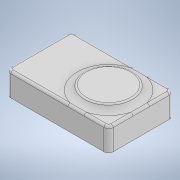
# Autodesk Inventor part: Black_Keyboard_Button
Saved by Autodesk Inventor 2021 (Build 250183000, 183)
## iProperties
Created: 2020-06-05
Part Number: Black_Keyboard_Button
Material: Generic
Document SubType Name: Modeling
Designer: ameli
Density: 1 g/cm^3
Appearance: Default
Author: ameli
Autodesk Inventor part; units mm, degrees
ref_plane "YZ Plane" through (0, 0, 0) normal (1, 0, 0) x (0, 1, 0)
ref_plane "XZ Plane" through (0, 0, 0) normal (0, 1, 0) x (-1, 0, 0)
ref_plane "XY Plane" through (0, 0, 0) normal (0, 0, 1) x (1, 0, 0)
sketch "Sketch1" plane through (0, 0, 0) normal (0, 1, 0) x (-1, 0, 0)
  line L0 (11, 7) -> (-11, 7)
  line L1 (-11, 7) -> (-11, -7)
  line L2 (-11, -7) -> (11, -7)
  line L3 (11, -7) -> (11, 7)
  point P0 (0, 0)
  dimension "d0" = 22
  dimension "d1" = 14
  dimension "d2" = 11
  dimension "d3" = 7
  constraints: 8 end point, 2 parallel, 1 horizontal, 1 perpendicular
  measures "d0" distance of L1.end L2.end
  measures "d1" distance of L2.end L0.start
  measures "d2" distance from line of point (0, 0) L3
  measures "d3" distance from line of point (0, 0) L2
extrude "Extrusion1" add sketch "Sketch1" along normal blind 5
sketch "Sketch2" plane through (0, 5, 0) normal (0, 1, 0) x (1, 0, 0)
  circle A0 centre (4, 0) radius 5
  line L0 (11, 7) -> (-11, 7) projected
  line L1 (11, -7) -> (11, 7) projected
  point P0 (0, 0)
  dimension "d6" = 10
  dimension "d7" = 7
  dimension "d8" = 7
  constraints: 1 centre point
  measures "d6" diameter of A0
  measures "d7" distance from line of L0 A0.centre
  measures "d8" distance from line of L1 A0.centre
extrude "Extrusion2" add sketch "Sketch2" along normal blind 1
fillet "Fillet1" radius 2 1 edges at (-1, 5, 0)
fillet "Fillet2" radius 1 4 edges at (11, 2.5, 7) (11, 2.5, -7) (-11, 2.5, 7) (-11, 2.5, -7)
fillet "Fillet3" radius 0.5 9 edges at (-1, 6, 0) (10.7071, 5, 6.7071) (11, 5, 0) (10.7071, 5, -6.7071) (0, 5, -7) (-10.7071, 5, -6.7071) (-11, 5, 0) (-10.7071, 5, 6.7071) (0, 5, 7)
sketch "Sketch3" plane through (0, 0, 0) normal (0, -1, 0) x (1, 0, 0)
  line L0 (-3, 3) -> (3, 3)
  line L1 (3, 3) -> (3, -3)
  line L2 (3, -3) -> (-3, -3)
  line L3 (-3, -3) -> (-3, 3)
  line L4 (-10, 7) -> (10, 7) projected
  point P0 (0, 0)
  dimension "d14" = 6
  dimension "d15" = 6
  dimension "d16" = 4
  dimension "d17" = 3
  constraints: 8 end point, 2 parallel, 1 horizontal, 1 perpendicular
  measures "d14" distance of L0.start L0.end
  measures "d15" distance of L0.end L1.end
  measures "d16" distance between parallel lines of L4 L0
  measures "d17" distance from line of point (0, 0) L1
extrude "Extrusion3" cut sketch "Sketch3" against normal blind 4.5
body "Solid1"
